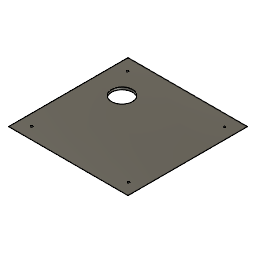
BBD - 200x200 mm (Autodesk Fusion 360 design; units mm, degrees)
part number: 2026-03-31-14-11-04-905
Autodesk Fusion 360 part; units mm, degrees
sketch "Esquisse1" plane through (0, 0, 0) normal (0, 0, 1) x (1, 0, 0)
  line L0 (0, 0) -> (200, 0)
  line L1 (200, 0) -> (200, 200)
  line L2 (200, 200) -> (0, 200)
  line L3 (0, 200) -> (0, 0)
  dimension "d18" = 200
  dimension "d19" = 200
  constraint horizontal L0
  constraint vertical L1
  constraint horizontal L2
  constraint vertical L3
  constraint coincident L0.start L3.end
  measures "d18" distance of L0 L2
  measures "d19" distance of L1 L3
extrude "Extrusion1" add sketch "Esquisse1" along normal blind 4
chamfer "Chanfrein1" distance 4 angle 45 1 faces at (66.6667, 133.3333, 0)
sketch "Esquisse2" plane through (0, 0, 4) normal (0, 0, 1) x (-1, 0, 0)
  circle A0 centre (-19, -180) radius 1.5
  circle A1 centre (-181, -180) radius 1.5
  circle A2 centre (-181, -20) radius 1.5
  circle A3 centre (-19, -20) radius 1.5
  line L0 (-200, 0) -> (-297.1716, 0) construction
  line L1 (0, -200) -> (-19, -180)
  line L2 (-200, -200) -> (-181, -180)
  line L3 (-200, -200) -> (-297.1716, -200) construction
  line L4 (0, -200) -> (0, 0)
  line L5 (0, 0) -> (-200, 0)
  line L6 (-200, 0) -> (-200, -200)
  line L7 (-200, -200) -> (0, -200)
  line L8 (-19, -180) -> (-19, -200)
  line L9 (-19, -180) -> (0, -180)
  line L10 (-181, -180) -> (-200, -180)
  line L11 (-181, -180) -> (-181, -200)
  line L12 (-181, -20) -> (-181, 0)
  line L13 (-181, -20) -> (-200, -20)
  line L14 (-19, -20) -> (-19, 0)
  line L15 (-19, -20) -> (0, -20)
  dimension "d10" = 3
  dimension "d11" = 3
  dimension "d12" = 3
  dimension "d13" = 3
  dimension "d37" = 20
  dimension "d38" = 19
  dimension "d39" = 19
  dimension "d40" = 20
  dimension "d41" = 19
  dimension "d42" = 20
  dimension "d43" = 19
  dimension "d44" = 20
  constraint horizontal L0
  constraint coincident A0.centre L1.end
  constraint horizontal L3
  constraint coincident A1.centre L2.end
  constraint coincident L0.start L5.end
  constraint coincident L2.start L3.start
  constraint coincident L1.start L4.start
  constraint coincident L7 L8.end
  constraint perpendicular L7 L8
  constraint coincident L4 L9.end
  constraint perpendicular L4 L9
  constraint coincident L6 L10.end
  constraint perpendicular L6 L10
  constraint coincident L7 L11.end
  constraint perpendicular L7 L11
  constraint coincident A2.centre L12.start
  constraint coincident L5 L12.end
  constraint perpendicular L5 L12
  constraint coincident L6 L13.end
  constraint perpendicular L6 L13
  constraint coincident A3.centre L14.start
  constraint coincident L5 L14.end
  constraint perpendicular L5 L14
  constraint coincident L4 L15.end
  constraint perpendicular L4 L15
  measures "d10" diameter of A0
  measures "d11" diameter of A1
  measures "d12" diameter of A2
  measures "d13" diameter of A3
  measures "d37" distance of A0.centre L8.end
  measures "d38" distance of A0.centre L9.end
  measures "d39" distance of A1.centre L10.end
  measures "d40" distance of A1.centre L11.end
  measures "d41" distance of A2.centre L13.end
  measures "d42" distance of A2.centre L12.end
  measures "d43" distance of A3.centre L15.end
  measures "d44" distance of A3.centre L14.end
extrude "Extrusion2" cut sketch "Esquisse2" against normal blind 14 contours A0 L8 L9 | A0 L1 L9 | A0 L1 L8 | A3 L14 L15 | A3 L14 L15 | A1 L10 L11 | A1 L2 L11 | A1 L2 L10 | A2 L12 L13 | A2 L12 L13
thread "Filetage1" "ISO Metric profile 4.0 M4x0.7 M4x0.7 6H" major diameter 4.1095 minor diameter 3.332 pitch 0.7 angle 60 resizes the face on face at (17.5464, 180.3701, 2.6667)
thread "Filetage2" "ISO Metric profile 4.0 M4x0.7 M4x0.7 6H" major diameter 4.1095 minor diameter 3.332 pitch 0.7 angle 60 resizes the face on face at (20.4925, 20.1494, 1.3333)
thread "Filetage3" "ISO Metric profile 4.0 M4x0.7 M4x0.7 6H" major diameter 4.1095 minor diameter 3.332 pitch 0.7 angle 60 resizes the face on face at (180.3157, 18.6652, 2.6667)
thread "Filetage4" "ISO Metric profile 4.0 M4x0.7 M4x0.7 6H" major diameter 4.1095 minor diameter 3.332 pitch 0.7 angle 60 resizes the face on face at (180.1244, 178.7821, 1.3333)
sketch "Esquisse3" plane through (0, 0, 4) normal (0, 0, 1) x (-1, 0, 0)
  circle A0 centre (-181, -180) radius 1.666
  circle A1 centre (-181, -20) radius 1.666
  circle A2 centre (-19, -180) radius 1.666
  circle A3 centre (-19, -20) radius 1.666
  line L0 (0, -200) -> (0, 0)
  line L1 (0, 0) -> (-200, 0)
  line L2 (-200, 0) -> (-200, -200)
  line L3 (-200, -200) -> (0, -200)
  circle A4 centre (-50, -140) radius 17.5
  point P0 (-50, -140)
  dimension "d28" = 50
  dimension "d29" = 60
  dimension "d30" = 35
  constraint coincident P0 A4.centre
  measures "d28" distance of L0 P0
  measures "d29" distance of L3 P0
  measures "d30" diameter of A4
extrude "Extrusion3" cut sketch "Esquisse3" against normal blind 10 contours A4
